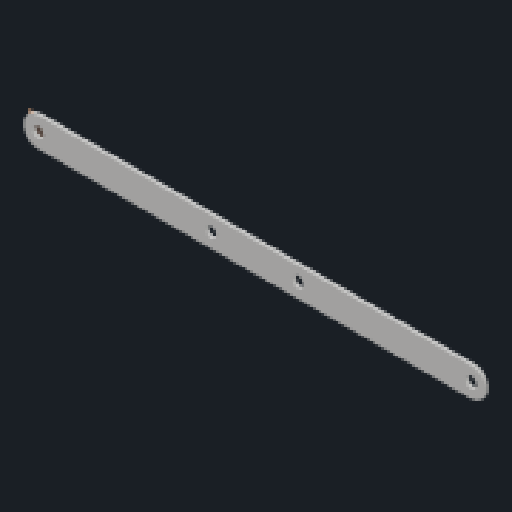
# Autodesk Inventor part: bottomSled
Saved by Autodesk Inventor 2023 (Build 270158000, 158)
## iProperties
Created: 2023-06-19
Part Number: bottomSled
Material: Generic
Document SubType Name: Modeling
Designer: reima
Density: 1 g/cm^3
Appearance: Default
Author: reima
Autodesk Inventor part; units mm, degrees
ref_plane "YZ Plane" through (0, 0, 0) normal (1, 0, 0) x (0, 1, 0)
ref_plane "XZ Plane" through (0, 0, 0) normal (0, 1, 0) x (-1, 0, 0)
ref_plane "XY Plane" through (0, 0, 0) normal (0, 0, 1) x (1, 0, 0)
ref_plane "Work Plane1" through (-190.5, 0, 0) normal (0, 0, 1) x (1, 0, 0)
sketch "Sketch1" plane through (-190.5, 0, 0) normal (0, 0, 1) x (1, 0, 0)
  circle A0 centre (0, 0) radius 2.4638 projected
  circle A1 centre (76.2, 0) radius 2.4638 projected
  circle A2 centre (114.3, 0) radius 2.4638 projected
  circle A3 centre (190.5, 0) radius 2.4638 projected
  circle A4 centre (0, 0) radius 6.35
  circle A5 centre (190.5, 0) radius 6.35
  line L0 (0, 6.35) -> (190.5, 6.35)
  line L1 (190.5, -6.35) -> (0, -6.35)
  point P0 (190.5, 0)
  dimension "d0" = 12.7
  dimension "d1" = 12.7
  constraints: 4 end point, 4 point on circle, 3 tangent, 2 centre point, 2 coincident, 1 horizontal
  measures "d0" diameter of A4
  measures "d1" diameter of A5
extrude "Extrusion1" add sketch "Sketch1" along normal blind 1.5875
body "Solid1"
